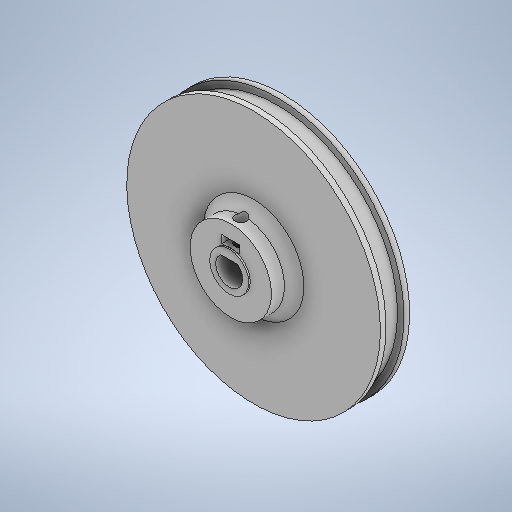
# Autodesk Inventor part: roue
Saved by Autodesk Inventor 2025.2 (Build 292293000, 293)
## iProperties
Created: 2025-03-27
Part Number: roue
Material: Générique
Document SubType Name: Modeling
Designer: enezl
Density: 1 g/cm^3
Appearance: Par défaut
Author: enezl
Autodesk Inventor part; units mm, degrees
ref_plane "YZ Plane" through (0, 0, 0) normal (1, 0, 0) x (0, 1, 0)
ref_plane "XZ Plane" through (0, 0, 0) normal (0, 1, 0) x (-1, 0, 0)
ref_plane "XY Plane" through (0, 0, 0) normal (0, 0, 1) x (1, 0, 0)
sketch "Esquisse1" plane through (0, 0, 0) normal (1, 0, 0) x (0, 1, 0)
  line L0 (37, -9) -> (37, 0) construction
  line L1 (0, 7.5) -> (6, 7.5)
  line L2 (12.5, 7) -> (12.5, 0)
  line L3 (0, 7.5) -> (0, -9)
  line L4 (0, 31.5501) -> (0, -31.5501)
  line L5 (37, -4.5) -> (0, -4.5) construction
  line L6 (12.5, 0) -> (39, 0)
  line L7 (39, 0) -> (39, -1.75)
  line L8 (39, -1.75) -> (37, -1.75)
  line L9 (37, -1.75) -> (37, -7.25)
  line L10 (0, -9) -> (39, -9)
  line L11 (39, -9) -> (39, -7.25)
  line L12 (39, -7.25) -> (37, -7.25)
  line L13 (12.5, 7) -> (6, 7)
  line L14 (6, 7) -> (6, 7.5)
  point P0 (0, 0)
  point P1 (6, 7.25)
  dimension "d1" = 9
  dimension "d4" = 0
  dimension "d5" = 74
  dimension "d6" = 25
  dimension "d20" = 2
  dimension "d21" = 2.75
  dimension "d31" = 16.5
  dimension "d32" = 6
  dimension "d33" = 0.5
  constraints: 30 end point, 6 perpendicular, 5 point on line, 3 midpoint, 3 symmetric about line, 2 horizontal, 2 vertical, 1 collinear, 1 other
  measures "d1" distance of L0.end L0.start
  measures "d4" distance between parallel lines of L3 L4
  measures "d5" diameter of L0 L4
  measures "d6" diameter of L2 L4
  measures "d20" distance of L7.end L8.end
  measures "d21" distance between parallel lines of L5 L8
  measures "d31" distance between parallel lines of L10 L1
  measures "d32" distance from line of L3 point (6, 7.25)
  measures "d33" distance between parallel lines of L13 L1
revolve "Révolution1" add sketch "Esquisse1" angle 360 about axis through (0, 0, 31.5501) along (0, 0, -1)
sketch "Esquisse2" plane through (0, 0, 0) normal (0, 1, 0) x (-1, 0, 0)
  circle A0 centre (0, 4) radius 1.75
  line L0 (-12.5, 7) -> (12.5, 7) projected
  point P0 (0, 0)
  dimension "d11" = 3.5
  dimension "d12" = 3
  constraints: 1 centre point
  measures "d11" diameter of A0
  measures "d12" distance from line of L0 A0.centre
extrude "Extrusion1" cut sketch "Esquisse2" along normal through all
sketch "Esquisse3" plane through (0, 0, 7) normal (0, 0, 1) x (1, 0, 0)
  line L0 (-2.75, 8.2) -> (2.75, 8.2)
  line L1 (2.75, 8.2) -> (2.75, 5.8)
  line L2 (2.75, 5.8) -> (-2.75, 5.8)
  line L3 (-2.75, 5.8) -> (-2.75, 8.2)
  line L4 (-2.75, 8.2) -> (2.75, 5.8) construction
  line L5 (2.75, 8.2) -> (-2.75, 5.8) construction
  line L6 (0, 7) -> (0, 0) construction
  point P0 (0, 0)
  dimension "d15" = 5.5
  dimension "d16" = 2.4
  dimension "d17" = 7
  constraints: 14 end point, 2 midpoint, 2 parallel, 1 horizontal, 1 perpendicular, 1 vertical
  measures "d15" distance of L0.start L0.end
  measures "d16" distance between parallel lines of L2 L0
  measures "d17" distance of L6.start L6.end
extrude "Extrusion2" cut sketch "Esquisse3" against normal blind 6
chamfer "Chanfrein1" distance 3 angle 45 1 edges at (0, -12.5, 0)
sketch "Esquisse4" plane through (0, 0, 7.5) normal (0, 0, 1) x (1, 0, 0)
  arc A0 (-2.6424, 3.2) -> (2.6424, 3.2) centre (0, 0) ccw
  line L0 (-2.6424, 3.2) -> (2.6424, 3.2)
  point P0 (0, 0)
  dimension "d27" = 8.3
  dimension "d28" = 3.2
  constraints: 2 end point, 2 point on circle, 1 centre point, 1 coincident, 1 horizontal
  measures "d27" diameter of A0
  measures "d28" distance from line of point (0, 0) L0
extrude "Extrusion3" cut sketch "Esquisse4" against normal through all
